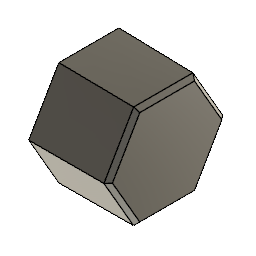
DoubleHook (Autodesk Fusion 360 archive; units mm, degrees)
design "SmallHexagonAssymetric"
Autodesk Fusion 360 part; units mm, degrees
sketch "HexagonBase" plane through (0, 0, 0) normal (1, 0, 0) x (0, 1, 0)
  line L0 (3.8394, 0) -> (7.6788, 6.65)
  line L1 (7.6788, 6.65) -> (3.8394, 13.3)
  line L2 (3.8394, 13.3) -> (-3.8394, 13.3)
  line L3 (-3.8394, 13.3) -> (-7.6788, 6.65)
  line L4 (-7.6788, 6.65) -> (-3.8394, 0)
  line L5 (-3.8394, 0) -> (3.8394, 0)
  line L6 (1.75, 0) -> (22.5, 0)
  point P0 (0, 6.65)
  dimension "d3" = 13.3
  constraint collinear L5 L6
  constraint midpoint origin L5
  measures "d3" distance of L2 L5
ref_plane "WorkPlane1" through (10, 0, 0) normal (1, 0, 0) x (0, 1, 0)
sketch "HexagonTip" plane through (10, 0, 0) normal (1, 0, 0) x (0, 1, 0)
  line L0 (3.7816, 0) -> (7.5633, 6.55)
  line L1 (7.5633, 6.55) -> (3.7816, 13.1)
  line L2 (3.7816, 13.1) -> (-3.7816, 13.1)
  line L3 (-3.7816, 13.1) -> (-7.5633, 6.55)
  line L4 (-7.5633, 6.55) -> (-3.7816, 0)
  line L5 (-3.7816, 0) -> (3.7816, 0)
  line L6 (1.75, 0) -> (22.5, 0)
  point P0 (0, 6.55)
  dimension "d5" = 13.1
  constraint collinear L5 L6
  constraint midpoint origin L5
  measures "d5" distance of L2 L5
loft "Loft1" add profiles "HexagonBase", "HexagonTip" section 1 section 2
chamfer "Chamfer1" distance 0.5 angle 45 6 edges at (10, 0, 13.1) (10, 5.6725, 9.825) (10, -5.6725, 9.825) (10, -5.6725, 3.275) (10, 0, 0) (10, 5.6725, 3.275)
equation "SmallHexagonInnerDiameter = 13.4 mm - 0.1 mm"
equation "d3 = SmallHexagonInnerDiameter"
equation "d5 = SmallHexagonInnerDiameter - 0.2 mm"
